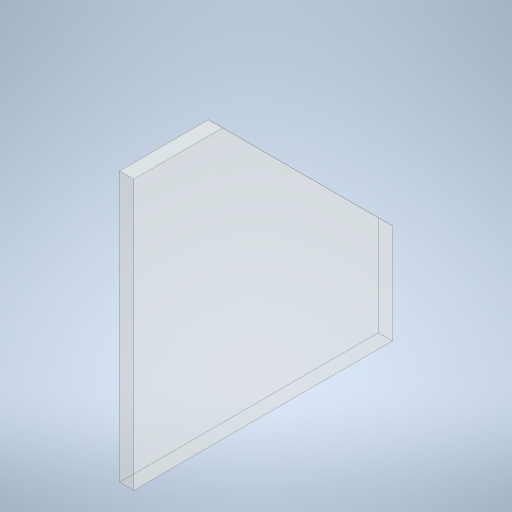
# Autodesk Inventor part: Wall_Between_Attic_Room_And_Stairwell
Saved by Autodesk Inventor 2024 (Build 280153000, 153)
## iProperties
Created: 2023-05-20
Part Number: Wall_Between_Attic_Room_And_Stairwell
Material: Wood (Southern Pine)
Document SubType Name: Modeling
Designer: Tom
Density: 0.420735 g/cm^3
Appearance: Clear
Author: Tom
Autodesk Inventor part; units mm, degrees
ref_plane "YZ Plane" through (0, 0, 0) normal (1, 0, 0) x (0, 1, 0)
ref_plane "XZ Plane" through (0, 0, 0) normal (0, 1, 0) x (-1, 0, 0)
ref_plane "XY Plane" through (0, 0, 0) normal (0, 0, 1) x (1, 0, 0)
sketch "Sketch1" plane through (0, 0, 0) normal (1, 0, 0) x (0, 1, 0)
  line L0 (0, 0) -> (2438.4, 0)
  line L1 (2438.4, 0) -> (2438.4, -800.1)
  line L2 (2438.4, -800.1) -> (914.4, -2324.1)
  line L3 (914.4, -2324.1) -> (0, -2324.1)
  line L4 (0, -2324.1) -> (0, 0)
  line L5 (2419.35, -792.2092) -> (2419.35, 0)
  line L6 (19.05, 0) -> (19.05, -2305.05)
  line L7 (19.05, -2305.05) -> (906.5092, -2305.05)
  line L8 (906.5092, -2305.05) -> (2419.35, -792.2092)
  dimension "d0" = 2324.1
  dimension "d1" = 2438.4
  dimension "d2" = 914.4
  dimension "d3" = 135
  dimension "d6" = 19.05
  dimension "d7" = 19.05
  dimension "d8" = 19.05
  constraints: 18 end point, 3 perpendicular, 2 point on line, 1 horizontal, 1 parallel, 1 other
  measures "d0" distance of L3.end L0.start
  measures "d1" distance of L0.start L0.end
  measures "d2" distance of L2.end L3.end
  measures "d3" angle of L3 L2
  measures "d6" distance between parallel lines of L5 L1
  measures "d7" distance between parallel lines of L2 L8
  measures "d8" distance between parallel lines of L6 L4
extrude "Extrusion1" add sketch "Sketch1" along normal blind 127 contours L0 L5 L8 L7 L6
body "Solid1"
